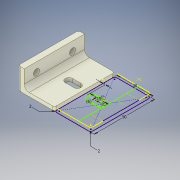
# Autodesk Inventor part: plate1
Saved by Autodesk Inventor 2019 (Build 230136000, 136)
## iProperties
Created: 2020-07-20
Part Number: plate1
Material: PC/ABS Plastic
Document SubType Name: Modeling
Designer: assman
Density: 0.357273 g/cm^3
Appearance: Smooth - White
Author: assman
Autodesk Inventor part; units mm, degrees
ref_plane "YZ Plane" through (0, 0, 0) normal (1, 0, 0) x (0, 1, 0)
ref_plane "XZ Plane" through (0, 0, 0) normal (0, 1, 0) x (-1, 0, 0)
ref_plane "XY Plane" through (0, 0, 0) normal (0, 0, 1) x (1, 0, 0)
sketch "Sketch1" plane through (0, 0, 0) normal (0, 1, 0) x (-1, 0, 0)
  line L0 (13, 25) -> (-13, 25)
  line L1 (-15, 23) -> (-15, -23)
  line L2 (-13, -25) -> (13, -25)
  line L3 (15, -23) -> (15, 23)
  line L4 (15, 25) -> (-15, -25) construction
  line L5 (-15, 25) -> (15, -25) construction
  line L6 (13, 0) -> (-2, 0) construction
  line L7 (9, 4) -> (2, 4)
  line L8 (2, -4) -> (9, -4)
  arc A0 (9, -4) -> (9, 4) centre (9, 0) ccw
  arc A1 (2, 4) -> (2, -4) centre (2, 0) ccw
  arc A2 (15, 23) -> (13, 25) centre (13, 23) ccw
  arc A3 (13, -25) -> (15, -23) centre (13, -23) ccw
  arc A4 (-15, -23) -> (-13, -25) centre (-13, -23) ccw
  arc A5 (-13, 25) -> (-15, 23) centre (-13, 23) ccw
  line L9 (9, -3) -> (2, -3)
  arc A6 (2, 3) -> (2, -3) centre (2, 0) ccw
  line L10 (2, 3) -> (9, 3)
  arc A7 (9, -3) -> (9, 3) centre (9, 0) ccw
  point P0 (0, 0)
  point P1 (5.5, 0)
  dimension "d0" = 30
  dimension "d1" = 50
  dimension "d2" = 15
  dimension "d3" = 8
  dimension "d4" = 2
  dimension "d5" = 2
  dimension "d6" = 2
  dimension "d32" = 1
  dimension "d33" = 6
  constraints: 24 end point, 18 point on circle, 12 tangent, 10 point on line, 8 centre point, 4 parallel, 3 midpoint, 2 equal radius, 2 perpendicular, 1 horizontal, 3 other
  measures "d0" distance of L5.end L4.end
  measures "d1" distance of L4.end L5.start
  measures "d2" distance of L6.start L6.end
  measures "d3" diameter of A1
  measures "d4" distance from line of L3 L6.start
  measures "d5" radius of A2
  measures "d6" radius of A5
  measures "d32" distance between parallel lines of L8 L9
  measures "d33" distance between parallel lines of L10 L9
extrude "Extrusion1" add sketch "Sketch1" along normal blind 3 contours A2 L3 A3 L2 A4 L1 A5 L0
sketch "Sketch2" plane through (0, 3, 0) normal (0, 1, 0) x (1, 0, 0)
  line L0 (5, 14.98) -> (15, 14.98) construction
  line L1 (15, 14.98) -> (15, -14.978)
  line L2 (15, -14.978) -> (5, -14.978) construction
  line L3 (5, -25) -> (5, 25)
  line L4 (15, -23) -> (15, 23) projected
  line L5 (13, 25) -> (-13, 25) projected
  line L6 (-13, -25) -> (13, -25) projected
  arc A0 (15, 23) -> (13, 25) centre (13, 23) ccw projected
  arc A1 (13, -25) -> (15, -23) centre (13, -23) ccw projected
  point P0 (0, 0)
  point P1 (10, 5.8278)
  constraints: 8 end point, 5 point on line, 2 parallel, 1 horizontal, 1 perpendicular
extrude "Extrusion2" add sketch "Sketch2" along normal blind 15
sketch "Sketch3" plane through (0, 18, 0) normal (0, 1, 0) x (1, 0, 0)
  point P0 (0, 0)
  point P1 (15, 14.98)
  point P2 (15, -14.978)
sketch "Sketch4" plane through (15, 0, 23) normal (1, 0, 0) x (0, 0, -1)
  line L0 (8.022, 18) -> (8.022, 3) construction
  line L1 (46, 3) -> (0, 3) construction
  line L2 (37.98, 18) -> (37.98, 3) construction
  point P0 (23, 0)
  point P1 (8.022, 10.5)
  point P2 (37.98, 10.5)
  constraints: 4 end point, 2 midpoint, 2 vertical, 1 point on line
hole "Hole1" at (15, 10.5, 14.978) at (15, 10.5, -14.98) direction (-1, 0, 0) diameter 5 end through all
sketch "Sketch5" plane through (0, 18, 0) normal (0, 1, 0) x (1, 0, 0)
  line L0 (5, 25) -> (5, -25) projected
  line L1 (5, -25) -> (13, -25) projected
  line L2 (13, 25) -> (5, 25) projected
  line L3 (10, -25) -> (10, 25)
  point P0 (0, 0)
  dimension "d27" = 5
  constraints: 2 end point, 2 point on line, 1 perpendicular
  measures "d27" distance between parallel lines of L0 L3
extrude "Extrusion3" cut sketch "Sketch5" against normal up to surface (15 mm away)
extrude "Extrusion4" add sketch "Sketch1" along normal up to surface (3 mm away) contours A0 L8 A1 L7
sketch "Sketch7" plane through (0, 3, 0) normal (0, 1, 0) x (1, 0, 0)
  line L0 (10, 25) -> (10, -25) projected
  arc A0 (-2, -3) -> (-2, 3) centre (-2, 0) ccw projected
  line L1 (-9, -3) -> (-2, -3) projected
  arc A1 (-9, 3) -> (-9, -3) centre (-9, 0) ccw projected
  line L2 (-2, 3) -> (-9, 3) projected
  line L3 (10, 25) -> (-13, 25) projected
  arc A2 (-13, 25) -> (-15, 23) centre (-13, 23) ccw projected
  line L4 (-15, 23) -> (-15, -23) projected
  arc A3 (-15, -23) -> (-13, -25) centre (-13, -23) ccw projected
  line L5 (-13, -25) -> (10, -25) projected
  line L6 (10, 25) -> (10, -25) projected
  line L7 (10, 22) -> (-15, 22)
  point P0 (0, 0)
  dimension "d37" = 3
  constraints: 2 end point, 2 point on line, 1 horizontal
  measures "d37" distance between parallel lines of L3 L7
extrude "Extrusion5" [suppressed]
sketch "Sketch8" plane through (13, 0, -25) normal (0, 0, -1) x (-1, 0, 0)
  line L0 (0, 0) -> (0, 18) construction
  line L1 (26, 0) -> (26, 3) construction
  line L2 (0, 3.0419) -> (26, 3.0419) construction
  line L3 (26, 3.0419) -> (26, 18) construction
  line L4 (26, 18) -> (0, 18) construction
  line L5 (0, 18) -> (0, 3.0419) construction
  line L6 (3, 16.771) -> (23, 16.771)
  line L7 (23, 16.771) -> (23, 4.271)
  line L8 (23, 4.271) -> (3, 4.271)
  line L9 (3, 4.271) -> (3, 16.771)
  line L10 (3, 16.771) -> (23, 4.271) construction
  line L11 (23, 16.771) -> (3, 4.271) construction
  circle A0 centre (13.0495, 10.521) radius 6.25
  line L12 (28, 0) -> (28, 3) projected
  point P0 (13, 0)
  point P1 (13, 10.521)
  point P2 (28, 18)
  dimension "d40" = 20
  dimension "d41" = 12.5
  dimension "d43" = 12.5
  dimension "d48" = 14.9505
  constraints: 20 end point, 4 parallel, 2 horizontal, 2 midpoint, 2 perpendicular, 1 centre point, 1 point on line
  measures "d40" distance of L7.end L8.end
  measures "d41" distance of L6.end L7.end
  measures "d43" diameter of A0
  measures "d48" distance from line of A0.centre L12
extrude "Extrusion6" [suppressed]
fillet "Fillet5" [suppressed]
fillet "Fillet6" radius 4 1 edges at (10, 3, 0)
mirror "Mirror2" about plane through (-15, 0, -23) normal (-1, 0, 0) remove original yes
body "Solid1"
